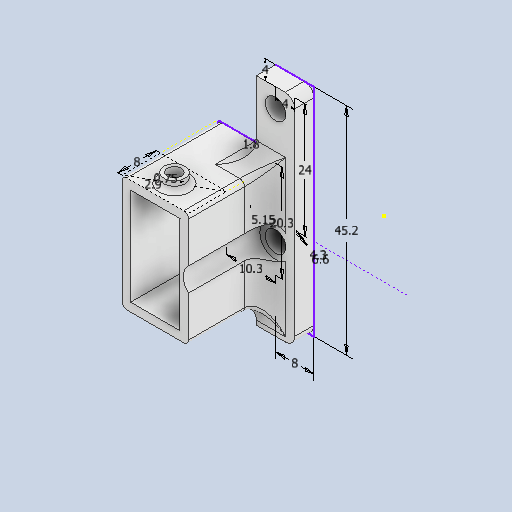
# Autodesk Inventor part: Part3
Saved by Autodesk Inventor 2023 (Build 270158000, 158)
## iProperties
Created: 2022-10-17
Part Number: Part3
Material: ABS Plastic
Document SubType Name: Modeling
Designer: Miner
Density: 1.06 g/cm^3
Appearance: Smooth - White
Author: Miner
Autodesk Inventor part; units mm, degrees
ref_plane "YZ Plane" through (0, 0, 0) normal (1, 0, 0) x (0, 1, 0)
ref_plane "XZ Plane" through (0, 0, 0) normal (0, 1, 0) x (-1, 0, 0)
ref_plane "XY Plane" through (0, 0, 0) normal (0, 0, 1) x (1, 0, 0)
sketch "Sketch1" plane through (0, 0, 0) normal (0, 0, 1) x (1, 0, 0)
  line L0 (-22.6, 22.6) -> (-14.6, 22.6)
  line L1 (-14.6, 22.6) -> (-14.6, -22.6)
  line L2 (-14.6, -22.6) -> (-22.6, -22.6)
  line L3 (-22.6, -22.6) -> (-22.6, 22.6)
  line L4 (5.4, -5.4) -> (-38.7938, -5.4) construction
  line L5 (-22.6, -5.4) -> (-27.75, -5.4) construction
  line L6 (-32.9, 4.75) -> (-22.6, 4.75)
  line L7 (-22.6, 4.75) -> (-22.6, -15.55)
  line L8 (-22.6, -15.55) -> (-32.9, -15.55)
  line L9 (-32.9, -15.55) -> (-32.9, 4.75)
  line L10 (-32.9, 4.75) -> (-22.6, -15.55) construction
  line L11 (-22.6, 4.75) -> (-32.9, -15.55) construction
  line L12 (-20.8, 6.55) -> (-34.7, 6.55)
  line L13 (-34.7, 6.55) -> (-34.7, -17.35)
  line L14 (-34.7, -17.35) -> (-20.8, -17.35)
  line L15 (-20.8, -17.35) -> (-20.8, 6.55)
  line L16 (-22.6, 22.6) -> (-22.6, 18.6) construction
  line L17 (-22.6, 18.6) -> (-18.6, 18.6) construction
  line L18 (-18.6, 18.6) -> (-18.6, -5.4) construction
  circle A0 centre (-18.6, -5.4) radius 3.3
  circle A1 centre (-18.6, -5.4) radius 2.15
  point P0 (-22.6, 6.55)
  point P1 (-22.6, -17.35)
  point P2 (-20.8, -2.9403)
  point P3 (-20.8, -7.8597)
  dimension "d0" = 8
  dimension "d1" = 45.2
  dimension "d2" = 5.15
  dimension "d3" = 10.3
  dimension "d4" = 20.3
  dimension "d5" = 1.8
  dimension "d10" = 4
  dimension "d11" = 4
  dimension "d12" = 24
  dimension "d32" = 6.6
  dimension "d35" = 4.3
  constraints: 38 end point, 6 parallel, 5 perpendicular, 5 point on line, 4 coincident, 2 centre point, 2 horizontal, 2 midpoint, 3 other
  measures "d0" distance of L1.end L2.end
  measures "d1" distance of L0.end L1.end
  measures "d2" distance of L5.start L5.end
  measures "d3" distance of L7.end L8.end
  measures "d4" distance of L6.end L7.end
  measures "d5" distance between parallel lines of L6 L12
  measures "d10" distance of L0.start L16.end
  measures "d11" distance of L16.end L17.end
  measures "d12" distance of L17.end L18.end
  measures "d32" diameter of A0
  measures "d35" diameter of A1
extrude "Extrusion1" add sketch "Sketch1" along normal blind 20 contours L12 L15 A0 L14 L3 | L3 L6 L9 L8 L14 L13 L12 | L15 A0 picked at (-20.9741, -4.7782)
extrude "Extrusion2" add sketch "Sketch1" along normal blind 4 contours L0 L1 L2 L3 L14 L15 A0 L12 | A0 L15 | A1 picked at (-15.7123, -5.1492)
hole "Hole1" at (-18.6, 18.6, 0) at (-18.6, -5.4, 0) direction (0, 0, 1) diameter 4.3 depth 5 tip angle 118
fillet "Fillet1" radius 4.3 5 edges at (-20.8, -5.4, 4) (-21.7, 6.55, 4) (-21.7, -17.35, 4) (-22.6, 6.55, 2) (-22.6, -17.35, 2)
fillet "Fillet3" radius 1 8 edges at (-34.7, 6.55, 10) (-34.7, -17.35, 10) (-23.85, 6.55, 8.3) (-19.55, 10.85, 4) (-20.8, 6.55, 14.15) (-23.85, -17.35, 8.3) (-19.55, -21.65, 4) (-20.8, -17.35, 14.15)
sketch "Sketch2" plane through (-26.9, 6.55, 8.3) normal (0, 1, 0) x (1, 0, 0)
  line L0 (6.1, -11.7) -> (6.1, 0) construction
  line L1 (-7.8, 8.3) -> (-7.8, -11.7) construction
  line L2 (6.1, -11.7) -> (-7.8, -11.7) construction
  line L3 (-7.8, -11.7) -> (-7.8, -3.7) construction
  line L4 (-7.8, -3.7) -> (6.1, -3.7) construction
  line L5 (6.1, -3.7) -> (6.1, -11.7) construction
  line L6 (-7.8, -11.7) -> (6.1, -3.7) construction
  circle A0 centre (-0.85, -7.7) radius 1.45
  circle A1 centre (-0.85, -7.7) radius 2.2
  point P0 (26.9, 8.3)
  dimension "d23" = 8
  dimension "d24" = 2.9
  dimension "d25" = 0.75
  constraints: 10 end point, 2 centre point, 2 parallel, 1 horizontal, 1 midpoint, 1 perpendicular, 1 point on line
  measures "d23" distance of L2.end L3.end
  measures "d24" diameter of A0
  measures "d25" radial gap between concentric circles of A0 A1
extrude "Extrusion3" add sketch "Sketch2" along normal blind 2
fillet "Fillet4" radius 2 2 edges at (-14.6, 22.6, 2) (-14.6, -22.6, 2)
fillet "Fillet5" radius 1 1 edges at (-29.95, 6.55, 16)
extrude "Extrusion4" cut sketch "Sketch2" against normal blind 2 contours A0
extrude "Extrusion5" cut sketch "Sketch1" along normal blind 20 contours A0 L15 | L15 A0 | A1
extrude "Extrusion6" add sketch "Sketch1" along normal blind 4 contours A0 L15 picked at (-15.7123, -5.1492)
extrude "Extrusion7" add sketch "Sketch1" along normal blind 4 contours L15 A0 picked at (-20.9741, -4.7782)
body "Solid1"
